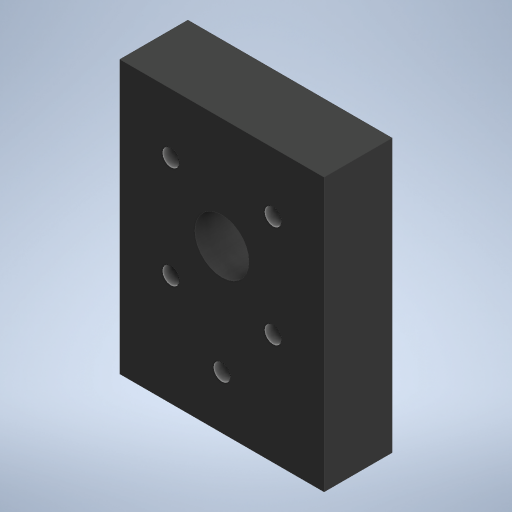
# Autodesk Inventor part: Motor Brace
Saved by Autodesk Inventor 2024 (Build 280153000, 153)
## iProperties
Created: 2025-01-21
Part Number: Motor Brace
Material: Generic
Document SubType Name: Modeling
Designer: Sven
Density: 1 g/cm^3
Appearance: Default
Author: Sven
Autodesk Inventor part; units mm, degrees
ref_plane "YZ Plane" through (0, 0, 0) normal (1, 0, 0) x (0, 1, 0)
ref_plane "XZ Plane" through (0, 0, 0) normal (0, 1, 0) x (-1, 0, 0)
ref_plane "XY Plane" through (0, 0, 0) normal (0, 0, 1) x (1, 0, 0)
sketch "Sketch1" plane through (0, 0, 0) normal (0, 0, 1) x (1, 0, 0)
  line L0 (-19.05, 25.4) -> (19.05, 25.4)
  line L1 (19.05, 25.4) -> (19.05, -25.4)
  line L2 (19.05, -25.4) -> (-19.05, -25.4)
  line L3 (-19.05, -25.4) -> (-19.05, 25.4)
  point P0 (0, 0)
  point P1 (19.05, 0)
  point P2 (0, 25.4)
  dimension "d0" = 38.1
  dimension "d1" = 50.8
  constraints: 8 end point, 2 midpoint, 2 parallel, 1 horizontal, 1 horizontal alignment, 1 perpendicular, 1 vertical alignment
  measures "d0" distance of L0.start L0.end
  measures "d1" distance of L0.end L1.end
extrude "Extrusion1" add sketch "Sketch1" along normal blind 12.7
sketch "Sketch2" plane through (0, 0, 12.7) normal (0, 0, 1) x (1, 0, 0)
  circle A0 centre (0, 4.7625) radius 5.05
  line L0 (19.05, 25.4) -> (-19.05, 25.4) projected
  circle A1 centre (0, -15.5575) radius 1.5875
  line L1 (0, 4.7625) -> (44.8131, 4.7625) construction
  line L2 (0, 4.7625) -> (0, 52.3228) construction
  circle A2 centre (9.525, 14.2875) radius 1.5875
  circle A3 centre (-9.525, 14.2875) radius 1.5875
  circle A4 centre (9.525, -4.7625) radius 1.5875
  circle A5 centre (-9.525, -4.7625) radius 1.5875
  point P0 (0, 0)
  dimension "d4" = 20.6375
  dimension "d5" = 10.1
  dimension "d8" = 3.175
  dimension "d9" = 20.32
  dimension "d11" = 3.175
  dimension "d12" = 9.525
  dimension "d13" = 9.525
  constraints: 6 centre point, 4 end point, 3 symmetric about line, 2 vertical alignment, 1 horizontal, 1 vertical, 3 other
  measures "d4" distance from line of L0 L1.start
  measures "d5" diameter of A0
  measures "d8" diameter of A1
  measures "d9" distance of A1.centre L1.start
  measures "d11" diameter of A2
  measures "d12" distance from line of L1 A2.centre
  measures "d13" distance from line of L2 A2.centre
extrude "Extrusion2" cut sketch "Sketch2" against normal up to surface (12.7 mm away)
body "Solid1"
